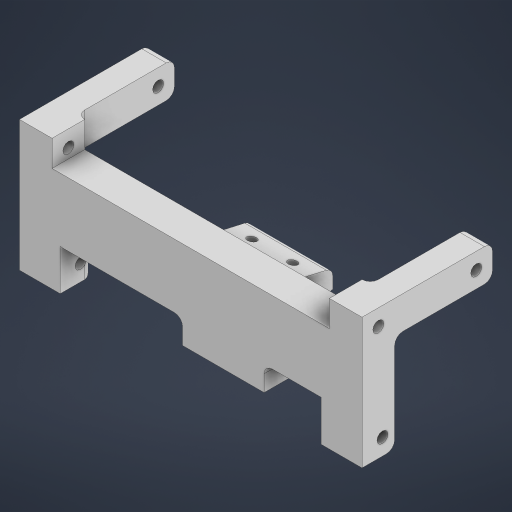
# Autodesk Inventor part: pto piston mount
Saved by Autodesk Inventor 2024 (Build 280153000, 153)
## iProperties
Created: 2024-03-30
Part Number: pto piston mount
Material: Generic
Document SubType Name: Modeling
Designer: Andrew
Density: 1 g/cm^3
Appearance: Default
Author: Andrew
Autodesk Inventor part; units mm, degrees
ref_plane "YZ Plane" through (0, 0, 0) normal (1, 0, 0) x (0, 1, 0)
ref_plane "XZ Plane" through (0, 0, 0) normal (0, 1, 0) x (-1, 0, 0)
ref_plane "XY Plane" through (0, 0, 0) normal (0, 0, 1) x (1, 0, 0)
sketch "Sketch1" plane through (0, 0, 0) normal (1, 0, 0) x (0, 1, 0)
  line L0 (0, 0) -> (38.1, 0)
  circle A0 centre (38.1, 0) radius 2.1336
  line L1 (38.1, 0) -> (38.1, -38.1)
  circle A1 centre (38.1, -38.1) radius 2.1336
  line L2 (0, 0) -> (-6.35, 0)
  line L3 (-6.35, 0) -> (-6.35, 6.35)
  line L4 (38.1, 0) -> (44.45, 0)
  line L5 (38.1, -38.1) -> (38.1, -44.45)
  line L6 (38.1, -44.45) -> (31.75, -44.45)
  line L7 (-6.35, 6.35) -> (44.45, 6.35)
  line L8 (44.45, 6.35) -> (44.45, -44.45)
  line L9 (44.45, -44.45) -> (38.1, -44.45)
  line L10 (-6.35, 0) -> (-6.35, -6.35)
  line L11 (-6.35, -6.35) -> (31.75, -6.35)
  line L12 (31.75, -6.35) -> (31.75, -44.45)
  line L13 (0, 0) -> (0, -1.6002)
  circle A2 centre (0, -1.6002) radius 2.1336
  dimension "d0" = 38.1
  dimension "d1" = 4.2672
  dimension "d2" = 38.1
  dimension "d3" = 4.2672
  dimension "d5" = 6.35
  dimension "d6" = 6.35
  dimension "d7" = 6.35
  dimension "d8" = 6.35
  dimension "d9" = 6.35
  dimension "d10" = 6.35
  dimension "d17" = 1.6002
  dimension "d18" = 4.2672
  constraints: 28 end point, 5 perpendicular, 4 coincident, 4 horizontal, 4 vertical, 3 centre point, 1 collinear
  measures "d0" distance of L0.start L0.end
  measures "d1" diameter of A0
  measures "d2" distance of L1.start L1.end
  measures "d3" diameter of A1
  measures "d5" distance of L2.start L2.end
  measures "d6" distance of L2.end L3.end
  measures "d7" distance of L1.start L4.end
  measures "d8" distance of L5.start L5.end
  measures "d9" distance of L5.end L6.end
  measures "d10" distance of L2.end L10.end
  measures "d17" distance of L2.start L13.end
  measures "d18" diameter of A2
extrude "Extrusion1" add sketch "Sketch1" along normal blind 6.35 contours A2 L2 L3 L7 L8 L4 A0 L0 | L0 A0 L1 A1 L5 L6 L12 L11 L10 L2 A2 | L4 L8 L9 L5 A1 L1 A0
sketch "Sketch5" plane through (6.35, 0, 0) normal (1, 0, 0) x (0, 0, -1)
  line L0 (-6.35, 44.45) -> (-6.35, -6.35) projected
  line L1 (-6.35, -6.35) -> (6.35, -6.35) projected
  line L2 (6.35, -6.35) -> (6.35, 31.75) projected
  line L3 (44.45, 44.45) -> (-6.35, 44.45) projected
  circle A0 centre (0, 38.1) radius 2.1336 projected
  circle A1 centre (1.6002, 0) radius 2.1336 projected
  line L4 (6.35, 31.75) -> (6.35, 44.45)
  point P0 (0, 0)
  constraints: 2 end point, 1 perpendicular, 1 point on line
extrude "Extrusion4" add sketch "Sketch5" along normal blind 114.3
sketch "Sketch6" plane through (120.65, 0, 0) normal (1, 0, 0) x (0, 0, -1)
  line L0 (6.35, -6.35) -> (6.35, 44.45) projected
  line L1 (6.35, 44.45) -> (-6.35, 44.45) projected
  line L2 (-6.35, 44.45) -> (-6.35, -6.35) projected
  line L3 (-6.35, -6.35) -> (6.35, -6.35) projected
  circle A0 centre (1.6002, 0) radius 2.1336 projected
  circle A1 centre (0, 38.1) radius 2.1336 projected
  line L4 (6.35, 31.75) -> (44.45, 31.75) projected
  line L5 (44.45, 44.45) -> (6.35, 44.45) projected
  line L6 (44.45, 31.75) -> (6.35, 31.75)
  line L7 (6.35, 31.75) -> (6.35, 44.45)
  line L8 (6.35, 44.45) -> (44.45, 44.45)
  line L9 (44.45, 44.45) -> (44.45, 31.75)
  circle A2 centre (38.1, 38.1) radius 2.1336 projected
  circle A3 centre (38.1, 38.1) radius 2.1336
  point P0 (0, 0)
  constraints: 8 end point, 2 parallel, 1 centre point, 1 coincident, 1 horizontal, 1 perpendicular
extrude "Extrusion5" add sketch "Sketch6" along normal blind 6.35
sketch "Sketch7" plane through (0, -6.35, -6.35) normal (0, 0, -1) x (-1, 0, 0)
  line L0 (0, 0) -> (-127, 0) projected
  line L1 (-120.65, 38.1) -> (-114.3, 38.1)
  line L2 (-6.35, 38.1) -> (-12.7, 38.1)
  line L3 (-114.3, 38.1) -> (-12.7, 38.1)
  line L4 (-12.7, 38.1) -> (-12.7, 0)
  line L5 (-12.7, 0) -> (-114.3, 0)
  line L6 (-114.3, 0) -> (-114.3, 38.1)
  line L7 (-114.3, 0) -> (-114.3, 15.875)
  line L8 (-114.3, 15.875) -> (-12.7, 15.875)
  point P0 (0, 6.35)
  point P1 (-114.3, 0)
  dimension "d23" = 6.35
  dimension "d26" = 15.875
  constraints: 16 end point, 3 point on line, 2 horizontal, 2 parallel, 2 perpendicular
  measures "d23" distance of L2.start L2.end
  measures "d26" distance of L5.end L7.end
extrude "Extrusion7" cut sketch "Sketch7" against normal through all contours L0 L6 L8 L4
sketch "Sketch11" plane through (127, 0, 0) normal (1, 0, 0) x (0, 0, -1)
  line L0 (6.35, -6.35) -> (6.35, 31.75) projected
  circle A0 centre (1.6002, 0) radius 2.1336 projected
  line L1 (1.6002, 0) -> (1.6002, 15.875)
  line L2 (1.6002, 15.875) -> (20.3454, 15.875)
  circle A1 centre (20.3454, 15.875) radius 5.588
  line L3 (6.35, -6.35) -> (6.35, 31.75) projected
  circle A2 centre (20.3454, 15.875) radius 12.7
  line L4 (20.3454, 28.575) -> (6.35, 31.75)
  line L5 (20.3454, 3.175) -> (6.35, 0)
  line L6 (20.3454, 28.575) -> (20.3454, 21.463)
  line L7 (20.3454, 10.287) -> (20.3454, 3.175)
  point P0 (0, 0)
  point P1 (6.35, 0)
  dimension "d38" = 15.875
  dimension "d39" = 18.7452
  dimension "d40" = 11.176
  dimension "d41" = 25.4
  constraints: 12 end point, 4 point on circle, 2 centre point, 2 coincident, 2 point on line, 2 vertical, 1 collinear, 1 horizontal
  measures "d38" distance of L1.start L1.end
  measures "d39" distance of L1.end L2.end
  measures "d40" diameter of A1
  measures "d41" diameter of A2
extrude "Extrusion11" add sketch "Sketch11" against normal blind 66.675 contours L0 L2 A2 L5 | L0 L4 A2 L2 | A2 L2 A1 L7 | A2 L6 A1 L2
sketch "Sketch12" plane through (127, 0, 0) normal (1, 0, 0) x (0, 0, -1)
  line L0 (6.35, -6.35) -> (6.35, 0) projected
  line L1 (6.35, 0) -> (20.3454, 3.175) projected
  line L2 (20.3454, 3.175) -> (20.3454, 10.287) projected
  arc A0 (20.3454, 21.463) -> (20.3454, 10.287) centre (20.3454, 15.875) ccw projected
  line L3 (20.3454, 21.463) -> (20.3454, 28.575) projected
  line L4 (20.3454, 28.575) -> (6.35, 31.75) projected
  line L5 (6.35, 31.75) -> (6.35, 9.525) projected
  line L6 (6.35, 31.75) -> (6.35, 0)
  point P0 (0, 0)
  constraints: 2 end point, 1 collinear
extrude "Extrusion12" cut sketch "Sketch12" against normal blind 34.925
sketch "Sketch13" plane through (60.325, 0, -6.35) normal (0, 0, 1) x (1, 0, 0)
  line L0 (31.75, 0) -> (31.75, 9.525) projected
  line L1 (31.75, 9.525) -> (0, 9.525) projected
  line L2 (0, 0) -> (0, 9.525) projected
  line L3 (31.75, 0) -> (0, 0) projected
  point P0 (-60.325, 0)
extrude "Extrusion13" add sketch "Sketch13" along normal up to surface (12.7 mm away)
sketch "Sketch14" plane through (60.325, 0, 6.35) normal (0, -1, 0) x (1, 0, 0)
  line L0 (31.75, -12.7) -> (0, -12.7) projected
  line L1 (0, -12.7) -> (31.75, -12.7)
  line L2 (15.875, -12.7) -> (0, -12.7)
  line L3 (15.875, -12.7) -> (31.75, -12.7)
  line L4 (23.8125, -12.7) -> (23.8125, -19.05)
  line L5 (7.9375, -12.7) -> (7.9375, -19.05)
  circle A0 centre (7.9375, -19.05) radius 1.778
  circle A1 centre (23.8125, -19.05) radius 1.778
  point P0 (-60.325, -6.35)
  dimension "d48" = 3.556
  dimension "d49" = 3.556
  constraints: 10 end point, 3 collinear, 3 midpoint, 2 centre point, 2 coincident, 2 vertical
  measures "d48" diameter of A0
  measures "d49" diameter of A1
extrude "Extrusion14" cut sketch "Sketch14" against normal through all
fillet "Fillet1" radius 3.175 21 edges at (120.65, -6.35, -6.35) (6.35, -6.35, -6.35) (3.175, 31.75, -44.45) (3.175, 44.45, -44.45) (3.175, 31.75, -6.35) (123.825, 31.75, -6.35) (123.825, 31.75, -44.45) (123.825, 44.45, -44.45) (6.35, 38.1, -6.35) (120.65, 38.1, -6.35) (60.325, 20.6375, -6.35) (76.2, 31.75, -6.35) (92.075, 20.6375, -6.35) (103.1875, 9.525, -6.35) (36.5125, 9.525, -6.35) (12.7, 1.5875, -6.35) (114.3, 1.5875, -6.35) (92.075, 9.525, 0) (60.325, 9.525, 0) (76.2, 3.175, -20.3454) (76.2, 28.575, -20.3454)
sketch "Sketch15" plane through (0, -3.175, -6.35) normal (0, 0, -1) x (-1, 0, 0)
  line L0 (-117.475, 31.75) -> (-117.475, 47.625) projected
  line L1 (-57.15, 37.4604) -> (-95.25, 37.4604) projected
  line L2 (-9.525, 47.625) -> (-9.525, 31.75) projected
  line L3 (-9.525, 47.625) -> (-117.475, 47.625) projected
  line L4 (-117.475, 47.625) -> (-9.525, 47.625)
  line L5 (-9.525, 47.625) -> (-9.525, 37.4604)
  line L6 (-9.525, 37.4604) -> (-117.475, 37.4604)
  line L7 (-117.475, 37.4604) -> (-117.475, 47.625)
  point P0 (0, 3.175)
  constraints: 8 end point, 2 parallel, 1 horizontal, 1 perpendicular, 1 point on line
extrude "Extrusion15" cut sketch "Sketch15" against normal through all
sketch "Sketch16" plane through (127, 0, 0) normal (1, 0, 0) x (0, 0, -1)
  circle A0 centre (38.1, 38.1) radius 2.1336 projected
  circle A1 centre (0, 38.1) radius 2.1336 projected
  circle A2 centre (1.6002, 0) radius 2.1336 projected
  arc A3 (44.45, 41.275) -> (41.275, 44.45) centre (41.275, 41.275) ccw projected
  line L0 (41.275, 44.45) -> (-6.35, 44.45) projected
  line L1 (-6.35, 44.45) -> (-6.35, -6.35) projected
  line L2 (-6.35, -6.35) -> (3.175, -6.35) projected
  arc A4 (3.175, -6.35) -> (6.35, -3.175) centre (3.175, -3.175) ccw projected
  line L3 (6.35, -3.175) -> (6.35, 28.575) projected
  arc A5 (9.525, 31.75) -> (6.35, 28.575) centre (9.525, 28.575) ccw projected
  line L4 (9.525, 31.75) -> (41.275, 31.75) projected
  arc A6 (41.275, 31.75) -> (44.45, 34.925) centre (41.275, 34.925) ccw projected
  line L5 (44.45, 34.925) -> (44.45, 41.275) projected
  point P0 (0, 0)
extrude "Extrusion16" add sketch "Sketch16" along normal blind 3.175
sketch "Sketch17" plane through (0, 0, 0) normal (-1, 0, 0) x (0, 0, 1)
  circle A0 centre (0, 38.1) radius 2.1336 projected
  circle A1 centre (-1.6002, 0) radius 2.1336 projected
  circle A2 centre (-38.1, 38.1) radius 2.1336 projected
  arc A3 (-41.275, 44.45) -> (-44.45, 41.275) centre (-41.275, 41.275) ccw projected
  line L0 (-44.45, 34.925) -> (-44.45, 41.275) projected
  arc A4 (-44.45, 34.925) -> (-41.275, 31.75) centre (-41.275, 34.925) ccw projected
  line L1 (-9.525, 31.75) -> (-41.275, 31.75) projected
  arc A5 (-6.35, 28.575) -> (-9.525, 31.75) centre (-9.525, 28.575) ccw projected
  line L2 (-6.35, -3.175) -> (-6.35, 28.575) projected
  arc A6 (-6.35, -3.175) -> (-3.175, -6.35) centre (-3.175, -3.175) ccw projected
  line L3 (6.35, -6.35) -> (-3.175, -6.35) projected
  line L4 (6.35, 44.45) -> (6.35, -6.35) projected
  line L5 (-41.275, 44.45) -> (6.35, 44.45) projected
  point P0 (0, 0)
extrude "Extrusion17" add sketch "Sketch17" along normal blind 3.175
body "Solid1"
